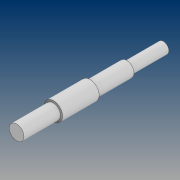
# Autodesk Inventor part: 02_Truc_01
Saved by Autodesk Inventor 2021 (Build 250183000, 183)
## iProperties
Created: 2024-03-11
Part Number: 02_Truc_01
Material: Generic
Document SubType Name: Modeling
Designer: Admin
Density: 1 g/cm^3
Appearance: Default
Author: Admin
Autodesk Inventor part; units mm, degrees
ref_plane "YZ Plane" through (0, 0, 0) normal (1, 0, 0) x (0, 1, 0)
ref_plane "XZ Plane" through (0, 0, 0) normal (0, 1, 0) x (-1, 0, 0)
ref_plane "XY Plane" through (0, 0, 0) normal (0, 0, 1) x (1, 0, 0)
sketch "Sketch1" plane through (0, 0, 0) normal (1, 0, 0) x (0, 1, 0)
  line L0 (0, -32.1759) -> (0, 79.8241) construction
  line L1 (0, 63.8241) -> (4, 63.8241)
  line L2 (4, 63.8241) -> (4, 43.8241)
  line L3 (4, 43.8241) -> (5, 43.8241)
  line L4 (5, 43.8241) -> (5, 23.8241)
  line L5 (5, 23.8241) -> (4, 23.8241)
  line L6 (4, 23.8241) -> (4, 3.8241)
  line L7 (4, 3.8241) -> (3, 3.8241)
  line L8 (3, 3.8241) -> (3, -16.1759)
  line L9 (3, -16.1759) -> (0, -16.1759)
  line L10 (0, 63.8241) -> (0, -16.1759)
  point P0 (0, 0)
  dimension "d0" = 3
  dimension "d1" = 80
  dimension "d2" = 60
  dimension "d3" = 20
  dimension "d4" = 4
  dimension "d5" = 5
  constraints: 20 end point, 7 perpendicular, 3 point on line, 2 vertical, 1 collinear, 1 horizontal
  measures "d0" distance between parallel lines of L0 L8
  measures "d1" distance between parallel lines of L1 L9
  measures "d2" distance between parallel lines of L7 L1
  measures "d3" distance of L3.end L4.end
  measures "d4" distance between parallel lines of L10 L2
  measures "d5" distance between parallel lines of L10 L4
revolve "Revolution1" add sketch "Sketch1" angle 360 about axis through (0, 0, 63.8241) along (0, 0, -1)
body "Solid1"
